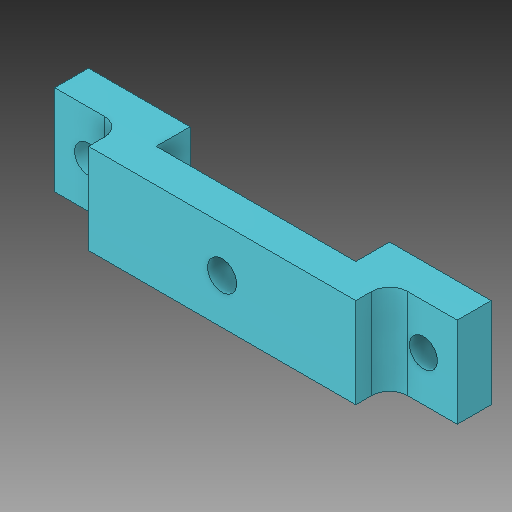
# Autodesk Inventor part: LowerSpringMount
Saved by Autodesk Inventor 2018.2 (Build 222227000, 227)
## iProperties
Created: 2018-03-24
Part Number: LowerSpringMount
Material: Generic
Document SubType Name: Modeling
Designer: MIABo
Density: 1 g/cm^3
Appearance: Default
Mass: 1.97507 g
Surface Area: 16.0965 cm^2
Volume: 1.97507 cm^3
Author: MIABo
## iProperties of the stored document LowerSpringMountRearBracket_3DPrint.ipt
Created: 2018-03-25
Part Number: LowerSpringMountRearBracket_3DPrint
Material: Generic
Document SubType Name: Modeling
Designer: MIABo
Density: 1 g/cm^3
Appearance: Default
Author: MIABo
Autodesk Inventor part; units mm, degrees
ref_plane "YZ Plane" through (0, 0, 0) normal (1, 0, 0) x (0, 1, 0)
ref_plane "XZ Plane" through (0, 0, 0) normal (0, 1, 0) x (-1, 0, 0)
ref_plane "XY Plane" through (0, 0, 0) normal (0, 0, 1) x (1, 0, 0)
sketch "Sketch1" plane through (0, 0, 0) normal (0, 0, 1) x (1, 0, 0)
  line L0 (-11.2395, -5.08) -> (11.2395, -5.08)
  line L1 (11.2395, -5.08) -> (11.2395, 5.08)
  line L2 (11.2395, 5.08) -> (-11.2395, 5.08)
  line L3 (-11.2395, 5.08) -> (-11.2395, -5.08)
  line L4 (-11.2395, -5.08) -> (11.2395, 5.08) construction
  line L5 (11.2395, -5.08) -> (-11.2395, 5.08) construction
  point P0 (0, 0)
  dimension "d0" = 22.479
  dimension "d1" = 10.16
  constraints: 12 end point, 2 midpoint, 2 parallel, 1 horizontal, 1 perpendicular
  measures "d0" distance of L2.end L1.end
  measures "d1" distance of L1.end L0.end
extrude "Extrusion1" add sketch "Sketch1" along normal blind 3.81
sketch "Sketch2" plane through (0, 0, 3.81) normal (0, 0, 1) x (1, 0, 0)
  line L0 (11.2395, 5.08) -> (-11.2395, 5.08) projected
  line L1 (-11.2395, 5.08) -> (-15.0495, 5.08)
  line L2 (-15.0495, 5.08) -> (-15.0495, -5.08)
  line L3 (-15.0495, -5.08) -> (-11.2395, -5.08)
  line L4 (-11.2395, -5.08) -> (-11.2395, 5.08)
  line L5 (11.2395, -5.08) -> (11.2395, 5.08) projected
  line L6 (11.2395, 5.08) -> (15.0495, 5.08)
  line L7 (15.0495, 5.08) -> (15.0495, -5.08)
  line L8 (15.0495, -5.08) -> (11.2395, -5.08)
  line L9 (11.2395, -5.08) -> (11.2395, 5.08)
  point P0 (0, 0)
  dimension "d4" = 3.81
  dimension "d5" = 10.16
  dimension "d6" = 3.81
  constraints: 16 end point, 4 parallel, 2 horizontal, 2 perpendicular
  measures "d4" distance of L3.end L2.end
  measures "d5" distance of L2.end L1.end
  measures "d6" distance of L7.end L8.end
extrude "Extrusion2" add sketch "Sketch2" against normal blind 7.62
sketch "Sketch3" plane through (0, 0, -3.81) normal (0, 0, -1) x (-1, 0, 0)
  line L0 (-11.2395, -5.08) -> (-11.2395, 5.08) projected
  line L1 (-11.2395, 5.08) -> (-22.6695, 5.08)
  line L2 (-22.6695, 5.08) -> (-22.6695, -5.08)
  line L3 (-22.6695, -5.08) -> (-11.2395, -5.08)
  line L4 (-11.2395, -5.08) -> (-11.2395, 5.08)
  line L5 (11.2395, 5.08) -> (11.2395, -5.08) projected
  line L6 (11.2395, 5.08) -> (22.6695, 5.08)
  line L7 (22.6695, 5.08) -> (22.6695, -5.08)
  line L8 (22.6695, -5.08) -> (11.2395, -5.08)
  line L9 (11.2395, -5.08) -> (11.2395, 5.08)
  point P0 (0, 0)
  dimension "d9" = 11.43
  dimension "d10" = 10.16
  dimension "d11" = 11.43
  dimension "d12" = 10.16
  constraints: 16 end point, 4 parallel, 2 horizontal, 2 perpendicular
  measures "d9" distance of L3.end L2.end
  measures "d10" distance of L1.end L2.end
  measures "d11" distance of L7.end L8.end
  measures "d12" distance of L6.end L7.end
extrude "Extrusion3" add sketch "Sketch3" against normal blind 3.81
sketch "Sketch4" plane through (0, 0, 0) normal (0, 0, -1) x (-1, 0, 0)
  circle A0 centre (0, 0) radius 1.651
  dimension "d15" = 3.302
  constraints: 1 centre point, 1 coincident
  measures "d15" diameter of A0
extrude "Extrusion4" cut sketch "Sketch4" against normal through all
sketch "Sketch5" plane through (0, 0, 0) normal (0, 0, 1) x (1, 0, 0)
  line L0 (15.0495, -5.08) -> (22.6695, -5.08) projected
  line L1 (-22.6695, -5.08) -> (-15.0495, -5.08) projected
  line L2 (22.6695, -5.08) -> (22.6695, 5.08) projected
  line L3 (-22.6695, 5.08) -> (-22.6695, -5.08) projected
  point P0 (0, 0)
  point P1 (-18.8595, 0)
  point P2 (18.8595, 0)
  dimension "d18" = 5.08
  dimension "d19" = 5.08
  dimension "d20" = 3.81
  dimension "d21" = 3.81
  measures "d18" distance from line of L0 point (18.859, 0)
  measures "d19" distance from line of L1 point (-18.86, 0)
  measures "d20" distance from line of L2 point (18.859, 0)
  measures "d21" distance from line of L3 point (-18.86, 0)
hole "Hole1" at (-18.8595, 0, 0) at (18.8595, 0, 0) direction (0, 0, -1) diameter 3.175 end through all
fillet "Fillet1" radius 2.032 2 edges at (15.0495, 0, 0) (-15.0495, 0, 0)
body "Solid1"
